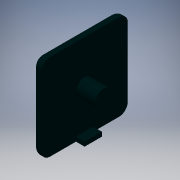
# Autodesk Inventor part: 18-813
Saved by Autodesk Inventor 2018 (Build 220105000, 105)
## iProperties
Created: 2006-02-19
Part Number: 18-813
Material: Glass Filled Nylon
Document SubType Name: Modeling
Designer: Autodesk, Inc.
Manufacturer: Standard
Standards Organization: Custom
Description: END CAP, 40 SERIES, 40x40
Catalog Web Link: http://www.parker.com/ead/cm1.asp?cmid=809
Vendor: PARKER IPS
Mass: 7.50143 g
Surface Area: 39.1851 cm^2
Volume: 6.63843 cm^3
Density: 1.13 g/cm^3
Appearance: Black (Plastic)
Author: Autodesk, Inc.
Autodesk Inventor part; units mm, degrees
ref_plane "YZ Plane" through (0, 0, 0) normal (1, 0, 0) x (0, 1, 0)
ref_plane "XZ Plane" through (0, 0, 0) normal (0, 1, 0) x (-1, 0, 0)
ref_plane "XY Plane" through (0, 0, 0) normal (0, 0, 1) x (1, 0, 0)
sketch "Sketch1" plane through (0, 0, 0) normal (0, 0, 1) x (1, 0, 0)
  line L0 (-20, 20) -> (20, 20)
  line L1 (20, 20) -> (20, -20)
  line L2 (20, -20) -> (-20, -20)
  line L3 (-20, -20) -> (-20, 20)
  point P0 (0, 0)
  point P1 (-20, 0)
  point P2 (0, 20)
  dimension "DimA" = 40
  dimension "DimB" = 40
  constraints: 8 end point, 2 midpoint, 2 parallel, 1 horizontal, 1 horizontal alignment, 1 perpendicular, 1 vertical alignment
  measures "DimA" distance of L0.start L0.end
  measures "DimB" distance of L2.end L0.start
extrude "Rectangluar End Cap" add sketch "Sketch1" along normal blind 4
sketch "Sketch6" plane through (0, 0, 4) normal (0, 0, 1) x (1, 0, 0)
  line L0 (-20, -20) -> (-20, 20) construction
  line L1 (20, -20) -> (-20, -20) construction
  circle A0 centre (0, 0) radius 3.9
  dimension "d37" = 20
  dimension "d38" = 20
  dimension "d39" = 7.8
  constraints: 1 centre point
  measures "d37" distance from line of A0.centre L0
  measures "d38" distance from line of A0.centre L1
  measures "d39" diameter of A0
extrude "Standard Post" add sketch "Sketch6" against normal blind 13
hole "Secure End Cap" [suppressed]
pattern_of_one "Rectangular Pattern3"
sketch "Sketch7" plane through (0, 0, 0) normal (0, 0, -1) x (-1, 0, 0)
  line L0 (-20, -20) -> (20, -20) construction
  line L1 (-4, -20) -> (4, -20)
  line L2 (4, -20) -> (4, -18)
  line L3 (4, -18) -> (-4, -18)
  line L4 (-4, -18) -> (-4, -20)
  line L5 (0, -18) -> (0, -20) construction
  point P0 (0, 0)
  dimension "d55" = 2
  dimension "d56" = 8
  constraints: 10 end point, 2 midpoint, 2 parallel, 2 point on line, 1 horizontal, 1 perpendicular
  measures "d55" distance of L3.end L1.start
  measures "d56" distance of L2.end L3.end
extrude "40x40 Orientation Tab" add sketch "Sketch7" along normal blind 4
fillet "Fillet5" radius 4 4 edges at (20, 20, 2) (-20, 20, 2) (-20, -20, 2) (20, -20, 2)
fillet "Fillet6" radius 2.5 8 edges at (-18.8284, -18.8284, 4) (0, -20, 4) (18.8284, -18.8284, 4) (20, 0, 4) (18.8284, 18.8284, 4) (0, 20, 4) (-18.8284, 18.8284, 4) (-20, 0, 4)
body "Solid1"
